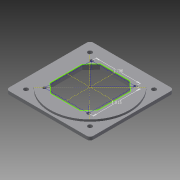
# Autodesk Inventor part: ka51a-instrument-mount
Saved by Autodesk Inventor 2015 (Build 190159000, 159)
## iProperties
Created: 2016-01-17
Part Number: ka51a-instrument-mount
Material: Generic
Document SubType Name: Modeling
Designer: bovine
Density: 1 g/cm^3
Appearance: Default
Author: bovine
Autodesk Inventor part; units mm, degrees
ref_plane "YZ Plane" through (0, 0, 0) normal (1, 0, 0) x (0, 1, 0)
ref_plane "XZ Plane" through (0, 0, 0) normal (0, 1, 0) x (-1, 0, 0)
ref_plane "XY Plane" through (0, 0, 0) normal (0, 0, 1) x (1, 0, 0)
sketch "Sketch1" plane through (0, 0, 0) normal (0, 1, 0) x (-1, 0, 0)
  line L0 (41.275, 41.275) -> (-41.275, 41.275)
  line L1 (-41.275, 41.275) -> (-41.275, -41.275)
  line L2 (-41.275, -41.275) -> (41.275, -41.275)
  line L3 (41.275, -41.275) -> (41.275, 41.275)
  circle A0 centre (0, 0) radius 44.45 construction
  circle A1 centre (0, 0) radius 39.6875
  line L4 (-41.275, 41.275) -> (41.275, -41.275) construction
  line L5 (41.275, 41.275) -> (-41.275, -41.275) construction
  circle A2 centre (31.4309, 31.4309) radius 2.159
  circle A3 centre (31.4309, -31.4309) radius 2.159
  circle A4 centre (-31.4309, 31.4309) radius 2.159
  circle A5 centre (-31.4309, -31.4309) radius 2.159
  point P0 (0, 0)
  point P1 (0, 0)
  point P2 (0, 0)
  dimension "d0" = 82.55
  dimension "d1" = 82.55
  dimension "d2" = 88.9
  dimension "d3" = 79.375
  dimension "d4" = 4.318
  dimension "d5" = 4.318
  dimension "d6" = 4.318
  dimension "d7" = 4.318
  constraints: 12 end point, 6 centre point, 4 coincident, 4 point on circle, 4 point on line, 2 midpoint, 2 parallel, 1 horizontal, 1 perpendicular
  measures "d0" distance of L2.end L1.end
  measures "d1" distance of L1.end L0.end
  measures "d2" diameter of A0
  measures "d3" diameter of A1
  measures "d4" diameter of A2
  measures "d5" diameter of A3
  measures "d6" diameter of A4
  measures "d7" diameter of A5
extrude "Extrusion1" add sketch "Sketch1" along normal blind 3.175 contours L3 L2 L1 L0 | A1
sketch "Sketch2" plane through (0, 3.175, 0) normal (0, 1, 0) x (1, 0, 0)
  circle A0 centre (0, 0) radius 39.0525
  circle A1 centre (0, 0) radius 39.6875 construction
  point P0 (0, 0)
  dimension "d10" = 78.105
  dimension "d17" = 79.375
  constraints: 2 centre point, 2 coincident
  measures "d10" diameter of A0
  measures "d17" diameter of A1
extrude "Extrusion2" add sketch "Sketch2" along normal blind 1.905
fillet "Fillet1" radius 3.175 1 edges at (41.275, 1.5875, 41.275)
fillet "Fillet2" radius 3.175 1 edges at (-41.275, 1.5875, 41.275)
fillet "Fillet3" radius 3.175 1 edges at (41.275, 1.5875, -41.275)
fillet "Fillet4" radius 3.175 1 edges at (-41.275, 1.5875, -41.275)
sketch "Sketch3" plane through (0, 5.08, 0) normal (0, 1, 0) x (1, 0, 0)
  line L0 (0, 24.765) -> (0, -24.765) construction
  line L1 (-23.3045, 0) -> (23.3045, 0) construction
  line L2 (-21.59, -23.0505) -> (21.59, -23.0505) construction
  line L3 (21.59, -23.0505) -> (21.59, 23.0505) construction
  line L4 (21.59, 23.0505) -> (-21.59, 23.0505) construction
  line L5 (-21.59, 23.0505) -> (-21.59, -23.0505) construction
  line L6 (-21.59, -23.0505) -> (21.59, 23.0505) construction
  line L7 (21.59, -23.0505) -> (-21.59, 23.0505) construction
  line L8 (-27.7495, -27.7495) -> (27.7495, 27.7495) construction
  line L9 (27.7495, -27.7495) -> (-27.7495, 27.7495) construction
  line L10 (-14.8242, 24.765) -> (14.1532, 24.765)
  line L11 (-14.8242, 24.765) -> (-23.3045, 15.7122)
  line L12 (23.3045, 16.1923) -> (23.3045, -15.7122)
  line L13 (23.3045, 16.1923) -> (14.1532, 24.765)
  line L14 (14.8242, -24.765) -> (-14.1532, -24.765)
  line L15 (14.8242, -24.765) -> (23.3045, -15.7122)
  line L16 (-23.3045, -16.1923) -> (-23.3045, 15.7122)
  line L17 (-23.3045, -16.1923) -> (-14.1532, -24.765)
  point P0 (0, 0)
  point P1 (0, 0)
  dimension "d20" = 43.18
  dimension "d21" = 46.101
  constraints: 36 end point, 6 parallel, 5 midpoint, 3 perpendicular, 2 horizontal, 1 coincident
  measures "d20" distance of L4.end L3.end
  measures "d21" distance of L3.end L2.end
extrude "Extrusion3" cut sketch "Sketch3" against normal through all
hole "Hole1" at (-21.59, 5.08, -23.0505) at (21.59, 5.08, 23.0505) at (21.59, 5.08, -23.0505) at (-21.59, 5.08, 23.0505) direction (0, -1, 0) diameter 3.175 end through all
body "Solid1"
